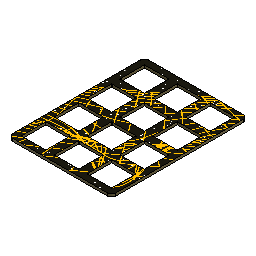
5128 MacroPad RP2040-Keyplate (Autodesk Fusion 360 design; units mm, degrees)
Autodesk Fusion 360 part; units mm, degrees
sketch "sketch 306" plane through (0, 0, 0) normal (0, 0, 1) x (1, 0, 0)
  line L0 (0, 76.2) -> (0, 2.54)
  arc A0 (0, 2.54) -> (2.54, 0) centre (2.54, 2.54) ccw
  line L1 (2.54, 0) -> (57.15, 0)
  arc A1 (57.15, 0) -> (59.69, 2.54) centre (57.15, 2.54) ccw
  line L2 (59.69, 2.54) -> (59.69, 76.2)
  arc A2 (59.69, 76.2) -> (57.15, 78.74) centre (57.15, 76.2) ccw
  line L3 (57.15, 78.74) -> (2.54, 78.74)
  arc A3 (2.54, 78.74) -> (0, 76.2) centre (2.54, 76.2) ccw
  line L4 (56.007, 75.057) -> (41.783, 75.057)
  line L5 (41.783, 75.057) -> (41.783, 60.833)
  line L6 (41.783, 60.833) -> (56.007, 60.833)
  line L7 (56.007, 60.833) -> (56.007, 75.057)
  line L8 (22.733, 75.057) -> (22.733, 60.833)
  line L9 (22.733, 60.833) -> (36.957, 60.833)
  line L10 (36.957, 60.833) -> (36.957, 75.057)
  line L11 (36.957, 75.057) -> (22.733, 75.057)
  line L12 (3.683, 75.057) -> (3.683, 60.833)
  line L13 (3.683, 60.833) -> (17.907, 60.833)
  line L14 (17.907, 60.833) -> (17.907, 75.057)
  line L15 (17.907, 75.057) -> (3.683, 75.057)
  line L16 (56.007, 56.007) -> (41.783, 56.007)
  line L17 (41.783, 56.007) -> (41.783, 41.783)
  line L18 (41.783, 41.783) -> (56.007, 41.783)
  line L19 (56.007, 41.783) -> (56.007, 56.007)
  line L20 (22.733, 56.007) -> (22.733, 41.783)
  line L21 (22.733, 41.783) -> (36.957, 41.783)
  line L22 (36.957, 41.783) -> (36.957, 56.007)
  line L23 (36.957, 56.007) -> (22.733, 56.007)
  arc A4 (3.937, 56.007) -> (3.683, 55.753) centre (3.937, 55.753) ccw
  line L24 (3.683, 55.753) -> (3.683, 41.783)
  line L25 (3.683, 41.783) -> (17.907, 41.783)
  line L26 (17.907, 41.783) -> (17.907, 56.007)
  line L27 (17.907, 56.007) -> (3.937, 56.007)
  line L28 (56.007, 22.733) -> (56.007, 36.957)
  line L29 (56.007, 36.957) -> (41.783, 36.957)
  line L30 (41.783, 36.957) -> (41.783, 22.733)
  line L31 (41.783, 22.733) -> (56.007, 22.733)
  arc A5 (22.987, 36.957) -> (22.733, 36.703) centre (22.987, 36.703) ccw
  line L32 (22.733, 36.703) -> (22.733, 22.733)
  line L33 (22.733, 22.733) -> (36.957, 22.733)
  line L34 (36.957, 22.733) -> (36.957, 36.957)
  line L35 (36.957, 36.957) -> (22.987, 36.957)
  line L36 (17.907, 22.733) -> (17.907, 36.957)
  line L37 (17.907, 36.957) -> (3.683, 36.957)
  line L38 (3.683, 36.957) -> (3.683, 22.733)
  line L39 (3.683, 22.733) -> (17.907, 22.733)
  line L40 (56.007, 17.907) -> (41.783, 17.907)
  line L41 (41.783, 17.907) -> (41.783, 3.683)
  line L42 (41.783, 3.683) -> (56.007, 3.683)
  line L43 (56.007, 3.683) -> (56.007, 17.907)
  arc A6 (22.987, 17.907) -> (22.733, 17.653) centre (22.987, 17.653) ccw
  line L44 (22.733, 17.653) -> (22.733, 3.683)
  line L45 (22.733, 3.683) -> (36.957, 3.683)
  line L46 (36.957, 3.683) -> (36.957, 17.907)
  line L47 (36.957, 17.907) -> (22.987, 17.907)
  line L48 (17.907, 3.683) -> (17.907, 17.907)
  line L49 (17.907, 17.907) -> (3.683, 17.907)
  line L50 (3.683, 17.907) -> (3.683, 3.683)
  line L51 (3.683, 3.683) -> (17.907, 3.683)
extrude "Board" add sketch "sketch 306" along normal blind 1.57 makes body 1 in component "Board"
sketch "sketch 765" plane through (0, 0, 0) normal (0, 0, 1) x (1, 0, 0)
  line L0 (0.01, -0.011) -> (59.787, -0.011)
  line L1 (59.787, -0.011) -> (59.787, 79.237)
  line L2 (59.787, 79.237) -> (0.01, 79.237)
  line L3 (0.01, 79.237) -> (0.01, -0.011)
extrude "MACROPAD_KEYPLATE" add sketch "sketch 765" along normal blind 0.1 separate body makes body 2 in component "MACROPAD_KEYPLATE"
component "PCB Component" placed x (1, 0, 0) y (0, 1, 0) z (0, 0, 1) at (0, 0, 0)
component "Board" placed x (1, 0, 0) y (0, 1, 0) z (0, 0, 1) at (0, 0, 0) in component "PCB Component"
component "MACROPAD_KEYPLATE" placed x (1, 0, 0) y (0, 1, 0) z (0, 0, 1) at (0, 0, 1.57) in component "PCB Component"
named bodies: "Board", "MACROPAD_KEYPLATE"
